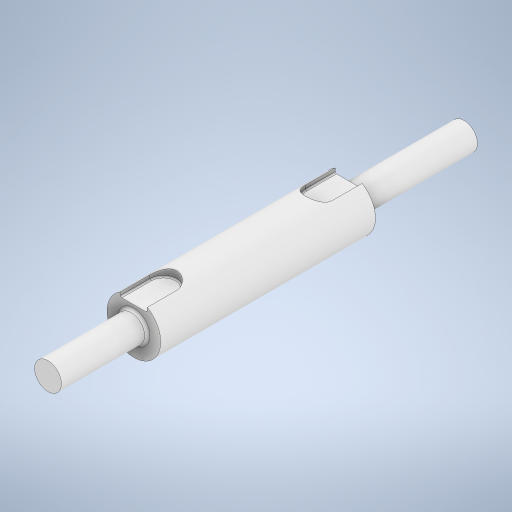
# Autodesk Inventor part: eje2
Saved by Autodesk Inventor 2024.3 (Build 283343000, 343)
## iProperties
Created: 2024-05-19
Part Number: eje2
Material: PBT Plastic
Document SubType Name: Modeling
Designer: USUARIO
Mass: 13.3759 g
Surface Area: 33.5597 cm^2
Volume: 10.2106 cm^3
Density: 1.31 g/cm^3
Appearance: Smooth - White
Author: USUARIO
Autodesk Inventor part; units mm, degrees
ref_plane "YZ Plane" through (0, 0, 0) normal (1, 0, 0) x (0, 1, 0)
ref_plane "XZ Plane" through (0, 0, 0) normal (0, 1, 0) x (-1, 0, 0)
sketch "Sketch1" plane through (0, 0, 0) normal (1, 0, 0) x (0, 1, 0)
  line L0 (0, 0) -> (5, 0)
  line L1 (5, 0) -> (5, -40)
  line L2 (5, -40) -> (0, -40)
  line L3 (0, -40) -> (0, 0)
  line L4 (0, 0) -> (2.5, 0)
  line L5 (2.5, 0) -> (2.5, 16)
  line L6 (2.5, 16) -> (0, 16)
  line L7 (0, 16) -> (0, 0)
  line L8 (0, -40) -> (2.5, -40)
  line L9 (2.5, -40) -> (2.5, -54)
  line L10 (2.5, -54) -> (0, -54)
  line L11 (0, -54) -> (0, -40)
  line L12 (0, -54) -> (2.5, -54)
  line L13 (2.5, -54) -> (2.5, -61.5)
  line L14 (2.5, -61.5) -> (0, -61.5)
  line L15 (0, -61.5) -> (0, -54)
  line L16 (0, 16) -> (2, 16)
  line L17 (0, 14) -> (0, 16)
  line L18 (0, 19.99) -> (0, -68.5807)
  point P0 (2.5, -40)
  dimension "d0" = 5
  dimension "d1" = 40
  dimension "d2" = 2.5
  dimension "d3" = 16
  dimension "d4" = 2.5
  dimension "d5" = 14
  dimension "d6" = 2.5
  dimension "d7" = 7.5
  constraints: 38 end point, 8 parallel, 5 horizontal, 4 perpendicular, 1 vertical
  measures "d0" distance of L1.end L2.end
  measures "d1" distance of L0.end L1.end
  measures "d2" distance of L6.end L5.end
  measures "d3" distance of L5.end L4.end
  measures "d4" distance of L9.end L10.end
  measures "d5" distance of L8.end L9.end
  measures "d6" distance of L13.end L14.end
  measures "d7" distance of L12.end L13.end
revolve "Revolution1" add sketch "Sketch1" angle 360 about axis through (0, 0, 19.99) along (0, 0, -1)
sketch "Sketch4" plane through (0, 0, 0) normal (0, 0, 1) x (1, 0, 0)
  circle A0 centre (0, 0) radius 5 construction
  line L0 (0, 5) -> (2.5, 5)
  line L1 (2.5, 5) -> (-2.5, 5)
  line L2 (-2.5, 5) -> (-2.5, 3.5)
  line L3 (-2.5, 3.5) -> (2.5, 3.5)
  line L4 (2.5, 3.5) -> (2.5, 5)
  point P0 (0, 0)
  dimension "d25" = 2.5
  dimension "d26" = 5
  dimension "d27" = 1.5
  constraints: 10 end point, 3 horizontal, 2 parallel, 1 perpendicular, 1 vertical alignment, 1 other
  measures "d25" distance of L0.start L0.end
  measures "d26" distance of L3.end L2.end
  measures "d27" distance of L2.end L1.end
extrude "Extrusion3" cut sketch "Sketch4" against normal blind 5.5
sketch "Sketch5" plane through (0, 0, -40) normal (0, 0, -1) x (-1, 0, 0)
  circle A0 centre (0, 0) radius 5 construction
  line L0 (0, 5) -> (2.5, 5)
  line L1 (-2.5, 4.3301) -> (-2.5, 3.5) projected
  line L2 (2.5, 5) -> (-2.5, 5)
  line L3 (-2.5, 5) -> (-2.5, 3.5)
  line L4 (-2.5, 3.5) -> (2.5, 3.5)
  line L5 (2.5, 3.5) -> (2.5, 5)
  point P0 (0, 0)
  dimension "d30" = 2.5
  dimension "d31" = 5
  dimension "d32" = 1.5
  constraints: 10 end point, 2 horizontal, 2 parallel, 1 perpendicular, 1 point on circle, 1 tangent
  measures "d30" distance of L0.start L0.end
  measures "d31" distance of L4.end L1.end
  measures "d32" distance of L1.end L2.end
extrude "Extrusion4" cut sketch "Sketch5" against normal blind 5.5
ref_plane "Work Plane1" through (0, 5, -20) normal (0, 1, 0) x (1, 0, 0)
sketch "Sketch6" plane through (0, 5, -20) normal (0, 1, 0) x (1, 0, 0)
  line L0 (2.5, -14.5) -> (-2.5, -14.5) projected
  circle A0 centre (0, -14.5) radius 2.5
  line L1 (-2.5, 14.5) -> (2.5, 14.5) projected
  circle A1 centre (0, 14.5) radius 2.5
  point P0 (0, -20)
  constraints: 2 horizontal alignment, 2 midpoint, 4 other
extrude "Extrusion5" cut sketch "Sketch6" against normal blind 1.5
fillet "Fillet2" radius 0.5 2 edges at (0, -2.5, 0) (0, -2.5, -40)
fillet "Fillet3" radius 0.25 6 edges at (0, 3.5, -8) (2.5, 3.5, -2.75) (-2.5, 3.5, -2.75) (0, 3.5, -32) (2.5, 3.5, -37.25) (-2.5, 3.5, -37.25)
body "Solid1"
